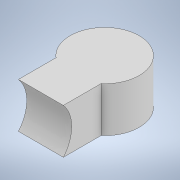
# Autodesk Inventor part: thigh
Saved by Autodesk Inventor 2020.2 (Build 242310000, 310)
## iProperties
Created: 2021-01-29
Part Number: thigh
Material: Generic
Document SubType Name: Modeling
Designer: DELL
Density: 1 g/cm^3
Appearance: Default
Mass: 601.418 g
Surface Area: 445.225 cm^2
Volume: 601.418 cm^3
Author: DELL
Autodesk Inventor part; units mm, degrees
ref_plane "YZ Plane" through (0, 0, 0) normal (1, 0, 0) x (0, 1, 0)
ref_plane "XZ Plane" through (0, 0, 0) normal (0, 1, 0) x (-1, 0, 0)
ref_plane "UCS1: YZ Plane" through (0, 0, 0) normal (1, 0, 0) x (0, 1, 0)
sketch "Sketch1" plane through (0, 0, 0) normal (1, 0, 0) x (0, 1, 0)
  circle A0 centre (0, 0) radius 30
  line L0 (-30, 0) -> (-30, -120)
  line L1 (-30, -120) -> (30, -120)
  line L2 (30, -120) -> (30, 0)
  circle A1 centre (0, 0) radius 46
  line L3 (0, -56) -> (15, -56)
  line L4 (15, -56) -> (15, -75)
  line L5 (15, -75) -> (0, -75)
  line L6 (0, -75) -> (0, -56)
  point P0 (30, -34.8712)
  point P1 (-30, -34.8712)
  point P2 (0, -46)
  dimension "d16" = 92
  dimension "d0" = 60
  dimension "d1" = 120
  dimension "d18" = 30
  dimension "d19" = 45
  dimension "d20" = 10
  dimension "d21" = 19
  constraints: 14 end point, 4 perpendicular, 2 coincident, 2 point on circle, 2 tangent, 2 vertical, 2 vertical alignment, 1 centre point, 1 horizontal, 3 other
  measures "d0" diameter of A0
  measures "d1" distance from line of point (0, 0) L1
  measures "d18" diameter of L4 L6
  measures "d19" distance between parallel lines of L1 L5
  measures "d20" distance of L3.start point (0, -46)
  measures "d21" distance of L3.end L4.end
extrude "Extrusion1" add sketch "Sketch1" along normal mid plane 60 contours L2 L1 L0 A1 | L3 L4 L5 L6
sketch "Sketch2" plane through (0, 0, 0) normal (0, 1, 0) x (-1, 0, 0)
  line L0 (-30, -120) -> (30, -120) projected
  circle A0 centre (0, -120) radius 46
  point P0 (0, 0)
  dimension "d4" = 92
  constraints: 1 centre point, 1 midpoint
  measures "d4" diameter of A0
extrude "Extrusion2" add sketch "Sketch2" along normal mid plane 60
ref_plane "Work Plane1" through (0, 0, -74) normal (0, 0, 1) x (1, 0, 0)
fillet "Fillet2" [suppressed]
equation "\"d4\" = d16"
body "Solid1"
